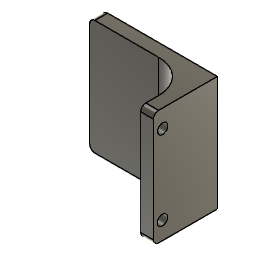
stand v1 (Autodesk Fusion 360 design; units mm, degrees)
Autodesk Fusion 360 part; units mm, degrees
sketch "Schizzo1" plane through (0, 0, 0) normal (0, 0, 1) x (1, 0, 0)
  line L0 (-8, 11.6314) -> (37, 11.6314)
  line L1 (37, 11.6314) -> (37, -13.3686)
  line L2 (37, -13.3686) -> (32, -13.3686)
  line L3 (32, -13.3686) -> (32, -6.3686)
  line L4 (-8, 11.6314) -> (-8, 6.6314)
  line L5 (-8, 6.6314) -> (19, 6.6314)
  arc A0 (32, -6.3686) -> (19, 6.6314) centre (19, -6.3686) ccw
  dimension "d1" = 5
  dimension "d2" = 5
  dimension "d3" = 45
  dimension "d4" = 25
  dimension "d5" = 13
  constraint horizontal L0
  constraint perpendicular L0 L1
  constraint perpendicular L1 L2
  constraint perpendicular L0 L3
  constraint perpendicular L0 L4
  constraint perpendicular L3 L5
  constraint tangent L3 A0
  constraint tangent L5 A0
  measures "d1" distance of L1.end L2.end
  measures "d2" distance of L0.start L4.end
  measures "d3" distance of L0.start L0.end
  measures "d4" distance of L0.end L1.end
  measures "d5" radius of A0
extrude "Estrusione1" add sketch "Schizzo1" along normal blind 45
fillet "Raccordo1" radius 2 4 edges at (-8, 9.1314, 0) (-8, 9.1314, 45) (34.5, -13.3686, 45) (34.5, -13.3686, 0)
sketch "Schizzo2" plane through (32, 0, 0) normal (-1, 0, 0) x (0, -1, 0)
  arc A0 (11.3686, 0) -> (13.3686, 2) centre (11.3686, 2) ccw
  line L0 (13.3686, 2) -> (13.3686, 43)
  arc A1 (13.3686, 43) -> (11.3686, 45) centre (11.3686, 43) ccw
  line L1 (11.3686, 45) -> (6.3686, 45)
  line L2 (6.3686, 45) -> (6.3686, 0)
  line L3 (6.3686, 0) -> (11.3686, 0)
  line L4 (9.8686, 7.0001) -> (6.3686, 7.0001) construction
  line L5 (9.8686, 7.0001) -> (13.3686, 7.0001) construction
  line L6 (9.7764, 37.9999) -> (6.3686, 37.9999) construction
  line L7 (9.7764, 37.9999) -> (13.1842, 37.9999) construction
  line L8 (9.7764, 37.9999) -> (9.7764, 45) construction
  line L9 (9.8686, 7.0001) -> (9.8686, 0) construction
  point P0 (9.8686, 7.0001)
  point P1 (9.7764, 37.9999)
  constraint coincident P0 L4.start
  constraint coincident L2 L4.end
  constraint perpendicular L2 L4
  constraint coincident L0 L5.end
  constraint perpendicular L0 L5
  constraint coincident P1 L6.start
  constraint coincident L2 L6.end
  constraint perpendicular L2 L6
  constraint perpendicular L0 L7
  constraint equal L4 L5
  constraint equal L6 L7
  constraint coincident L1 L8.end
  constraint perpendicular L1 L8
  constraint coincident L3 L9.end
  constraint perpendicular L3 L9
  constraint equal L8 L9
hole "Foratura1" at (32, -9.8686, 7.0001) at (32, -9.7764, 37.9999) direction (1, 0, 0) diameter 4 depth 11 tip angle 118 countersink diameter 6 countersink angle 90
sketch "Schizzo4" plane through (0, 11.6314, 0) normal (0, 1, 0) x (-1, 0, 0)
  arc A0 (8, 43) -> (6, 45) centre (6, 43) ccw
  line L0 (6, 45) -> (-37, 45)
  line L1 (-37, 45) -> (-37, 0)
  line L2 (-37, 0) -> (6, 0)
  arc A1 (6, 0) -> (8, 2) centre (6, 2) ccw
  line L3 (8, 2) -> (8, 43)
  circle A2 centre (-14.5, 22.5) radius 19.5
  dimension "d19" = 39
  dimension "d20" = 22.5
  dimension "d21" = 22.5
  dimension "d22" = 22.5
  dimension "d23" = 22.5
  measures "d19" diameter of A2
  measures "d20" distance of L0 A2.centre
  measures "d21" distance of L3 A2.centre
  measures "d22" distance of L1 A2.centre
  measures "d23" distance of L2 A2.centre
extrude "Estrusione2" cut sketch "Schizzo4" against normal blind 2.5 contours A2
fillet "Raccordo2" radius 0.5 1 edges at (32.6804, 11.6314, 29.5515)
